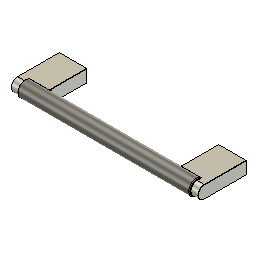
Hafele 115.70 Configurable (Autodesk Fusion 360 archive; units mm, degrees)
design "L148"
description: Handle
part number: 115.70.148
Autodesk Fusion 360 part; units mm, degrees
note: some values were not read from the file. Chosen so that the rebuilt part matches the saved one: which bodies a step acts on; which face or edge a step refers to.
sketch "Sketch1" plane through (0, 0, 0) normal (0, 0, 1) x (1, 0, 0)
  line L0 (74, 5) -> (-74, 5)
  line L1 (-74, 5) -> (-74, -5)
  line L2 (-74, -5) -> (74, -5)
  line L3 (74, -5) -> (74, 5)
  line L4 (74, 5) -> (-74, -5) construction
  line L5 (-74, 5) -> (74, -5) construction
  dimension "d2" = 148
  dimension "d3" = 10
  constraint horizontal L0
  constraint perpendicular L0 L1
  constraint parallel L0 L2
  constraint parallel L1 L3
  constraint coincident L4 origin
  constraint coincident L5 origin
  measures "d2" distance of L1.end L2.end
  measures "d3" distance of L0.end L1.end
sketch "Sketch2" plane through (0, 0, 0) normal (1, 0, 0) x (0, 0, -1)
  line L0 (0, 5) -> (-38, 5)
  line L1 (-38, 5) -> (-38, -5)
  line L2 (-38, -5) -> (0, -5)
  line L3 (0, -5) -> (0, 5)
  line L4 (0, 5) -> (0, -5)
  point P0 (0, 5)
  point P1 (0, -5)
  dimension "d4" = 38
  constraint horizontal L0
  constraint vertical L1
  constraint horizontal L2
  constraint vertical L3
  constraint coincident P0 L0.start
  constraint coincident P1 L2.end
  measures "d4" distance of L1 L4
extrude "Extrude1" add sketch "Sketch2" along normal mid plane 148 makes body 1
sketch "Sketch3" plane through (0, 5, 0) normal (0, 1, 0) x (-1, 0, 0)
  line L0 (74, 38) -> (-74, 38)
  line L1 (-74, 38) -> (-74, 0)
  line L2 (-74, 0) -> (74, 0)
  line L3 (74, 0) -> (74, 38)
  line L4 (74, 0) -> (52, 0)
  line L5 (52, 0) -> (52, 38)
  line L6 (52, 38) -> (74, 38)
  line L7 (74, 38) -> (74, 0)
  line L8 (-74, 0) -> (-52, 0)
  line L9 (-52, 0) -> (-52, 38)
  line L10 (-52, 38) -> (-74, 38)
  line L11 (-74, 38) -> (-74, 0)
  dimension "d7" = 22
  dimension "d8" = 22
  constraint horizontal L4
  constraint vertical L5
  constraint horizontal L6
  constraint vertical L7
  constraint coincident L0 L5.end
  constraint coincident L2.end L3.start
  constraint horizontal L8
  constraint vertical L9
  constraint horizontal L10
  constraint vertical L11
  constraint coincident L0 L9.end
  constraint coincident L1.end L2.start
  measures "d7" distance of L5 L7
  measures "d8" distance of L9 L11
extrude "Extrude2" cut sketch "Sketch3" against normal through all contours L0 L2 L5 L9 bodies 1 makes body 2 at (59.3333, -5, 25.3333)
fillet "Fillet1" radius 5 4 edges at (-63, 5, 38) (-63, -5, 38) (63, 5, 38) (63, -5, 38) on bodies 1 2
sketch "Sketch4" plane through (0, 0, 0) normal (0, 1, 0) x (1, 0, 0)
  line L0 (68, -39) -> (-68, -39)
  line L1 (-68, -39) -> (-68, -33)
  line L2 (-68, -33) -> (68, -33)
  line L3 (68, -33) -> (68, -39)
  line L4 (68, -39) -> (-68, -33) construction
  line L5 (-68, -39) -> (68, -33) construction
  line L6 (-74, -33) -> (-74, 0)
  line L7 (74, 0) -> (74, -33)
  line L8 (-41, -33) -> (-85, -33)
  point P0 (0, -36)
  dimension "d12" = 6
  dimension "d13" = 6
  dimension "d14" = 6
  constraint horizontal L0
  constraint perpendicular L0 L1
  constraint parallel L0 L2
  constraint parallel L1 L3
  constraint coincident L4 P0
  constraint coincident L5 P0
  constraint collinear L2 L8
  measures "d12" distance of L1 L6
  measures "d13" distance of L3 L7.end
  measures "d14" distance of L0 L2
revolve "Revolve1" cut sketch "Sketch4" angle 360 about axis through (-68, 0, 33) along (1, 0, 0) bodies 1 2
revolve "Revolve2" add sketch "Sketch4" angle 360 about axis through (-68, 0, 33) along (1, 0, 0) bodies 1 2
chamfer "Chamfer1" distance 0.2 angle 45 26 edges at (-52, 0, 27) (52, 0, 27) (-68, 5, 31.3422) (-68, 3.5358, 36.5358) (-68, 0, 38) (-68, -3.5358, 36.5358) (-68, -5, 31.3422) (-74, -5, 16.5005) (-52, -5, 14.8417) (-52, 5, 14.8417) (-74, 5, 16.5005) (68, -5, 31.3422) (68, -3.5358, 36.5358) (68, 0, 38) (68, 3.5358, 36.5358) (68, 5, 31.3422) (52, 5, 14.8417) (74, 5, 16.5005) (52, -5, 14.8417) (74, -5, 16.5005) (-74, 3.5358, 36.5358) (-74, 0, 38) (-74, -3.5358, 36.5358) (74, -3.5358, 36.5358) (74, 0, 38) (74, 3.5358, 36.5358) on bodies 1 2
fillet "Fillet2" radius 0.2 4 edges at (-60, 5, 29.6834) (-60, -5, 29.6834) (60, -5, 29.6834) (60, 5, 29.6834) on bodies 1
chamfer "Chamfer2" distance 0.5 angle 45 4 edges at (68, -5.1942, 36.0033) (-68, -5.1942, 36.0033) (68, 5.1942, 36.0033) (-68, 5.1942, 36.0033) on bodies 1
sketch "Sketch5" plane through (0, 0, 0) normal (0, 0, -1) x (-1, 0, 0)
  line L0 (-52.2, -5) -> (-52, -4.8)
  line L1 (-52, -4.8) -> (-52, 4.8)
  line L2 (-52, 4.8) -> (-52.2, 5)
  line L3 (-52.2, 5) -> (-73.8, 5)
  line L4 (-73.8, 5) -> (-74, 4.8)
  line L5 (-74, 4.8) -> (-74, -4.8)
  line L6 (-74, -4.8) -> (-73.8, -5)
  line L7 (-73.8, -5) -> (-52.2, -5)
  line L8 (-64, 0) -> (-62, 0) construction
  line L9 (-62, 0) -> (64, 0) construction
  line L10 (74, 4.8) -> (74, -4.8) construction
  dimension "d21" = 10
  dimension "d22" = 10
  constraint perpendicular L1 L8
  constraint perpendicular L1 L9
  measures "d21" distance of L5 L8.start
  measures "d22" distance of L9.end L10
hole "Hole1" at (64, 0, 0) at (-64, 0, 0) direction (0, 0, 1) diameter 3.332 depth 20 tip angle 118 countersink diameter 4.5 countersink angle 90 bodies 1
thread "Thread1" "ISO Metric profile 4.0 M4x0.7 M4x0.7 6H" thread offset 0 thread depth 7.4
sketch "Bolts" plane through (0, 0, 0) normal (0, 0, -1) x (-1, 0, 0)
  circle A0 centre (64, 0) radius 2.25
  line L0 (52, -4.8) -> (52.2, -5)
  line L1 (52.2, -5) -> (73.8, -5)
  line L2 (73.8, -5) -> (74, -4.8)
  line L3 (74, -4.8) -> (74, 4.8)
  line L4 (74, 4.8) -> (73.8, 5)
  line L5 (73.8, 5) -> (52.2, 5)
  line L6 (52.2, 5) -> (52, 4.8)
  line L7 (52, 4.8) -> (52, -4.8)
  line L8 (64, 0) -> (60.1135, 0)
  line L9 (60.1135, 0) -> (-64, 0) construction
  circle A1 centre (-64, 0) radius 2.25
  constraint parallel L5 L8
  constraint parallel L5 L9
  constraint coincident A0.centre L8.start
  constraint coincident L9.end A1.centre
equation "HandeLength = 148 mm"
equation "d2 = HandeLength"
equation "d5 = HandeLength"
equation "d8 = d7"
equation "d13 = d12"
equation "d22 = d21"

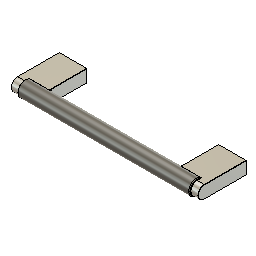
design "hafele 115.70 configurable handle"
description: Handle
part number: 115.70.148
Autodesk Fusion 360 part; units mm, degrees
sketch "Sketch1" plane through (0, 0, 0) normal (0, 0, 1) x (1, 0, 0)
  line L0 (74, 5) -> (-74, 5)
  line L1 (-74, 5) -> (-74, -5)
  line L2 (-74, -5) -> (74, -5)
  line L3 (74, -5) -> (74, 5)
  line L4 (74, 5) -> (-74, -5) construction
  line L5 (-74, 5) -> (74, -5) construction
  dimension "d2" = 148
  dimension "d3" = 10
  constraint horizontal L0
  constraint perpendicular L0 L1
  constraint parallel L0 L2
  constraint parallel L1 L3
  constraint coincident L4 origin
  constraint coincident L5 origin
  measures "d2" distance of L1.end L2.end
  measures "d3" distance of L0.end L1.end
sketch "Sketch2" plane through (0, 0, 0) normal (1, 0, 0) x (0, 0, -1)
  line L0 (0, 5) -> (-38, 5)
  line L1 (-38, 5) -> (-38, -5)
  line L2 (-38, -5) -> (0, -5)
  line L3 (0, -5) -> (0, 5)
  line L4 (0, 5) -> (0, -5)
  point P0 (0, 5)
  point P1 (0, -5)
  dimension "d4" = 38
  constraint horizontal L0
  constraint vertical L1
  constraint horizontal L2
  constraint vertical L3
  constraint coincident P0 L0.start
  constraint coincident P1 L2.end
  measures "d4" distance of L1 L4
extrude "Extrude1" add sketch "Sketch2" along normal mid plane 148 makes body 1
sketch "Sketch3" plane through (0, 5, 0) normal (0, 1, 0) x (-1, 0, 0)
  line L0 (74, 38) -> (-74, 38)
  line L1 (-74, 38) -> (-74, 0)
  line L2 (-74, 0) -> (74, 0)
  line L3 (74, 0) -> (74, 38)
  line L4 (74, 0) -> (52, 0)
  line L5 (52, 0) -> (52, 38)
  line L6 (52, 38) -> (74, 38)
  line L7 (74, 38) -> (74, 0)
  line L8 (-74, 0) -> (-52, 0)
  line L9 (-52, 0) -> (-52, 38)
  line L10 (-52, 38) -> (-74, 38)
  line L11 (-74, 38) -> (-74, 0)
  dimension "d7" = 22
  dimension "d8" = 22
  constraint horizontal L4
  constraint vertical L5
  constraint horizontal L6
  constraint vertical L7
  constraint coincident L0 L5.end
  constraint coincident L2.end L3.start
  constraint horizontal L8
  constraint vertical L9
  constraint horizontal L10
  constraint vertical L11
  constraint coincident L0 L9.end
  constraint coincident L1.end L2.start
  measures "d7" distance of L5 L7
  measures "d8" distance of L9 L11
extrude "Extrude2" cut sketch "Sketch3" against normal through all contours L0 L2 L5 L9 bodies 1 makes body 2 at (59.3333, -5, 25.3333)
fillet "Fillet1" radius 5 4 edges at (-63, 5, 38) (-63, -5, 38) (63, 5, 38) (63, -5, 38) on bodies 1 2
sketch "Sketch4" plane through (0, 0, 0) normal (0, 1, 0) x (1, 0, 0)
  line L0 (68, -39) -> (-68, -39)
  line L1 (-68, -39) -> (-68, -33)
  line L2 (-68, -33) -> (68, -33)
  line L3 (68, -33) -> (68, -39)
  line L4 (68, -39) -> (-68, -33) construction
  line L5 (-68, -39) -> (68, -33) construction
  line L6 (-74, -33) -> (-74, 0)
  line L7 (74, 0) -> (74, -33)
  line L8 (-41, -33) -> (-85, -33)
  point P0 (0, -36)
  dimension "d12" = 6
  dimension "d13" = 6
  dimension "d14" = 6
  constraint horizontal L0
  constraint perpendicular L0 L1
  constraint parallel L0 L2
  constraint parallel L1 L3
  constraint coincident L4 P0
  constraint coincident L5 P0
  constraint collinear L2 L8
  measures "d12" distance of L1 L6
  measures "d13" distance of L3 L7.end
  measures "d14" distance of L0 L2
revolve "Revolve1" cut sketch "Sketch4" angle 360 about axis through (-68, 0, 33) along (1, 0, 0) bodies 1 2
revolve "Revolve2" add sketch "Sketch4" angle 360 about axis through (-68, 0, 33) along (1, 0, 0) bodies 1 2
chamfer "Chamfer1" distance 0.2 angle 45 26 edges at (-52, 0, 27) (52, 0, 27) (-68, 5, 31.3422) (-68, 3.5358, 36.5358) (-68, 0, 38) (-68, -3.5358, 36.5358) (-68, -5, 31.3422) (-74, -5, 16.5005) (-52, -5, 14.8417) (-52, 5, 14.8417) (-74, 5, 16.5005) (68, -5, 31.3422) (68, -3.5358, 36.5358) (68, 0, 38) (68, 3.5358, 36.5358) (68, 5, 31.3422) (52, 5, 14.8417) (74, 5, 16.5005) (52, -5, 14.8417) (74, -5, 16.5005) (-74, 3.5358, 36.5358) (-74, 0, 38) (-74, -3.5358, 36.5358) (74, -3.5358, 36.5358) (74, 0, 38) (74, 3.5358, 36.5358) on bodies 1 2
fillet "Fillet2" radius 0.2 4 edges at (-60, 5, 29.6834) (-60, -5, 29.6834) (60, -5, 29.6834) (60, 5, 29.6834) on bodies 1
chamfer "Chamfer2" distance 0.5 angle 45 4 edges at (68, -5.1942, 36.0033) (-68, -5.1942, 36.0033) (68, 5.1942, 36.0033) (-68, 5.1942, 36.0033) on bodies 1
sketch "Sketch5" plane through (0, 0, 0) normal (0, 0, -1) x (-1, 0, 0)
  line L0 (-52.2, -5) -> (-52, -4.8)
  line L1 (-52, -4.8) -> (-52, 4.8)
  line L2 (-52, 4.8) -> (-52.2, 5)
  line L3 (-52.2, 5) -> (-73.8, 5)
  line L4 (-73.8, 5) -> (-74, 4.8)
  line L5 (-74, 4.8) -> (-74, -4.8)
  line L6 (-74, -4.8) -> (-73.8, -5)
  line L7 (-73.8, -5) -> (-52.2, -5)
  line L8 (-64, 0) -> (-62, 0) construction
  line L9 (-62, 0) -> (64, 0) construction
  line L10 (74, 4.8) -> (74, -4.8) construction
  dimension "d21" = 10
  dimension "d22" = 10
  constraint perpendicular L1 L8
  constraint perpendicular L1 L9
  measures "d21" distance of L5 L8.start
  measures "d22" distance of L9.end L10
hole "Hole1" at (64, 0, 0) at (-64, 0, 0) direction (0, 0, 1) diameter 3.332 depth 20 tip angle 118 countersink diameter 4.5 countersink angle 90 bodies 1
thread "Thread1" "ISO Metric profile 4.0 M4x0.7 M4x0.7 6H" thread offset 0 thread depth 7.4
sketch "Bolts" plane through (0, 0, 0) normal (0, 0, -1) x (-1, 0, 0)
  circle A0 centre (64, 0) radius 2.25
  line L0 (52, -4.8) -> (52.2, -5)
  line L1 (52.2, -5) -> (73.8, -5)
  line L2 (73.8, -5) -> (74, -4.8)
  line L3 (74, -4.8) -> (74, 4.8)
  line L4 (74, 4.8) -> (73.8, 5)
  line L5 (73.8, 5) -> (52.2, 5)
  line L6 (52.2, 5) -> (52, 4.8)
  line L7 (52, 4.8) -> (52, -4.8)
  line L8 (64, 0) -> (60.1135, 0)
  line L9 (60.1135, 0) -> (-64, 0) construction
  circle A1 centre (-64, 0) radius 2.25
  constraint parallel L5 L8
  constraint parallel L5 L9
  constraint coincident A0.centre L8.start
  constraint coincident L9.end A1.centre
equation "HandeLength = 148 mm"
equation "d2 = HandeLength"
equation "d5 = HandeLength"
equation "d8 = d7"
equation "d13 = d12"
equation "d22 = d21"
